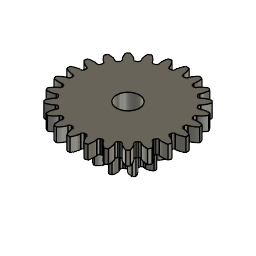
IntermediateGear1 (Autodesk Fusion 360 design; units mm, degrees)
part number: 2026-05-31-22-24-32-655
Autodesk Fusion 360 part; units mm, degrees
sketch "Base Circle" plane through (0, 0, 0) normal (0, 0, 1) x (1, 0, 0)
  circle A0 centre (0, 0) radius 1.9215
  circle A1 centre (0, 0) radius 1.25
  dimension "d49" = 2.5
  measures "d49" diameter of A1
extrude "Extrude9" add sketch "Base Circle" along normal blind 10 makes body 1
sketch "Gear Tooth" plane through (0, 0, 0) normal (0, 0, 1) x (1, 0, 0)
  spline S0 degree 5 poles (2.3146, -0.402) (2.3164, -0.4024) (2.3202, -0.403) (2.3258, -0.4036) (2.3334, -0.4042) (2.3429, -0.4044) (2.3525, -0.4042) (2.3621, -0.4039) (2.3717, -0.4033) (2.3814, -0.4027) (2.3911, -0.4021) (2.4007, -0.4013) (2.4104, -0.4003) (2.4202, -0.3992) (2.4299, -0.3979) (2.4396, -0.3964) (2.4494, -0.3947) (2.4592, -0.393) (2.469, -0.3911) (2.4788, -0.3892) (2.4886, -0.3871) (2.4984, -0.3849) (2.5082, -0.3826) (2.518, -0.3802) (2.5279, -0.3777) (2.5377, -0.3751) (2.5476, -0.3723) (2.5574, -0.3695) (2.5673, -0.3665) (2.5771, -0.3634) (2.587, -0.3603) (2.5968, -0.357) (2.6067, -0.3537) (2.6166, -0.3503) (2.6264, -0.3467) (2.6363, -0.3431) (2.6462, -0.3393) (2.656, -0.3355) (2.6659, -0.3316) (2.6757, -0.3276) (2.6856, -0.3235) (2.6954, -0.3193) (2.7053, -0.315) (2.7151, -0.3106) (2.7249, -0.3061) (2.7348, -0.3016) (2.7446, -0.2969) (2.7544, -0.2922) (2.7642, -0.2874) (2.774, -0.2825) (2.7838, -0.2775) (2.7936, -0.2724) (2.8034, -0.2673) (2.8131, -0.262) (2.8229, -0.2567) (2.8327, -0.2513) (2.8424, -0.2458) (2.8521, -0.2402) (2.8618, -0.2346) (2.8715, -0.2288) (2.8812, -0.223) (2.8909, -0.2171) (2.9006, -0.2111) (2.9102, -0.2051) (2.9199, -0.1989) (2.9295, -0.1927) (2.9391, -0.1864) (2.9487, -0.18) (2.9583, -0.1735) (2.9678, -0.167) (2.9774, -0.1604) (2.985, -0.155) (2.9907, -0.151) (2.9945, -0.1482) (2.9964, -0.1469) knots 0 0 0 0 0 0 0.01428571 0.02857143 0.04285714 0.05714286 0.07142857 0.08571429 0.1 0.11428571 0.12857143 0.14285714 0.15714286 0.17142857 0.18571429 0.2 0.21428571 0.22857143 0.24285714 0.25714286 0.27142857 0.28571429 0.3 0.31428571 0.32857143 0.34285714 0.35714286 0.37142857 0.38571429 0.4 0.41428571 0.42857143 0.44285714 0.45714286 0.47142857 0.48571429 0.5 0.51428571 0.52857143 0.54285714 0.55714286 0.57142857 0.58571429 0.6 0.61428571 0.62857143 0.64285714 0.65714286 0.67142857 0.68571429 0.7 0.71428571 0.72857143 0.74285714 0.75714286 0.77142857 0.78571429 0.8 0.81428571 0.82857143 0.84285714 0.85714286 0.87142857 0.88571429 0.9 0.91428571 0.92857143 0.94285714 0.95714286 0.97142857 0.98571429 1 1 1 1 1 1
  spline S1 degree 5 poles (2.3146, 0.402) (2.3164, 0.4024) (2.3202, 0.403) (2.3258, 0.4036) (2.3334, 0.4042) (2.3429, 0.4044) (2.3525, 0.4042) (2.3621, 0.4039) (2.3717, 0.4033) (2.3814, 0.4027) (2.3911, 0.4021) (2.4007, 0.4013) (2.4104, 0.4003) (2.4202, 0.3992) (2.4299, 0.3979) (2.4396, 0.3964) (2.4494, 0.3947) (2.4592, 0.393) (2.469, 0.3911) (2.4788, 0.3892) (2.4886, 0.3871) (2.4984, 0.3849) (2.5082, 0.3826) (2.518, 0.3802) (2.5279, 0.3777) (2.5377, 0.3751) (2.5476, 0.3723) (2.5574, 0.3695) (2.5673, 0.3665) (2.5771, 0.3634) (2.587, 0.3603) (2.5968, 0.357) (2.6067, 0.3537) (2.6166, 0.3503) (2.6264, 0.3467) (2.6363, 0.3431) (2.6462, 0.3393) (2.656, 0.3355) (2.6659, 0.3316) (2.6757, 0.3276) (2.6856, 0.3235) (2.6954, 0.3193) (2.7053, 0.315) (2.7151, 0.3106) (2.7249, 0.3061) (2.7348, 0.3016) (2.7446, 0.2969) (2.7544, 0.2922) (2.7642, 0.2874) (2.774, 0.2825) (2.7838, 0.2775) (2.7936, 0.2724) (2.8034, 0.2673) (2.8131, 0.262) (2.8229, 0.2567) (2.8327, 0.2513) (2.8424, 0.2458) (2.8521, 0.2402) (2.8618, 0.2346) (2.8715, 0.2288) (2.8812, 0.223) (2.8909, 0.2171) (2.9006, 0.2111) (2.9102, 0.2051) (2.9199, 0.1989) (2.9295, 0.1927) (2.9391, 0.1864) (2.9487, 0.18) (2.9583, 0.1735) (2.9678, 0.167) (2.9774, 0.1604) (2.985, 0.155) (2.9907, 0.151) (2.9945, 0.1482) (2.9964, 0.1469) knots 0 0 0 0 0 0 0.01428571 0.02857143 0.04285714 0.05714286 0.07142857 0.08571429 0.1 0.11428571 0.12857143 0.14285714 0.15714286 0.17142857 0.18571429 0.2 0.21428571 0.22857143 0.24285714 0.25714286 0.27142857 0.28571429 0.3 0.31428571 0.32857143 0.34285714 0.35714286 0.37142857 0.38571429 0.4 0.41428571 0.42857143 0.44285714 0.45714286 0.47142857 0.48571429 0.5 0.51428571 0.52857143 0.54285714 0.55714286 0.57142857 0.58571429 0.6 0.61428571 0.62857143 0.64285714 0.65714286 0.67142857 0.68571429 0.7 0.71428571 0.72857143 0.74285714 0.75714286 0.77142857 0.78571429 0.8 0.81428571 0.82857143 0.84285714 0.85714286 0.87142857 0.88571429 0.9 0.91428571 0.92857143 0.94285714 0.95714286 0.97142857 0.98571429 1 1 1 1 1 1
  arc A0 (2.9964, -0.1469) -> (2.9964, 0.1469) centre (0, 0) ccw
  line L0 (1.8833, -0.3271) -> (2.3146, -0.402)
  line L1 (1.8833, 0.3271) -> (2.3146, 0.402)
  line L2 (1.8833, -0.3271) -> (1.8833, 0.3271)
  point P0 (2.3614, -0.4039)
  point P1 (2.4092, -0.4004)
  point P2 (2.4574, -0.3933)
  point P3 (2.5061, -0.3831)
  point P4 (2.555, -0.3701)
  point P5 (2.6041, -0.3546)
  point P6 (2.6534, -0.3365)
  point P7 (2.7027, -0.3161)
  point P8 (2.752, -0.2934)
  point P9 (2.8012, -0.2684)
  point P10 (2.8504, -0.2412)
  point P11 (2.8993, -0.2119)
  point P12 (2.948, -0.1804)
  point P13 (2.3614, 0.4039)
  point P14 (2.4092, 0.4004)
  point P15 (2.4574, 0.3933)
  point P16 (2.5061, 0.3831)
  point P17 (2.555, 0.3701)
  point P18 (2.6041, 0.3546)
  point P19 (2.6534, 0.3365)
  point P20 (2.7027, 0.3161)
  point P21 (2.752, 0.2934)
  point P22 (2.8012, 0.2684)
  point P23 (2.8504, 0.2412)
  point P24 (2.8993, 0.2119)
  point P25 (2.948, 0.1804)
extrude "Extrude10" add sketch "Gear Tooth" along normal blind 10 bodies 1
fillet "Fillet4" radius 0.2 2 edges at (1.8932, -0.3288, 5) (1.8932, 0.3288, 5) on bodies 1
pattern_circular "C-Pattern4" count 10 over 360 about axis through (0, 0, 0) along (0, 0, 1) of "Extrude10", "Fillet4"
sketch "Diametrial Pitch Circle" plane through (0, 0, 0) normal (0, 0, 1) x (1, 0, 0)
  circle A0 centre (0, 0) radius 2.5 construction
extrude "Extrude11" cut 1 faces at (1.7096, 0, 10) along direction (0, 0, -1) blind 8 on bodies 1 bodies 1
sketch "Base Circle (1)" plane through (0, 0, 0) normal (0, 0, 1) x (1, 0, 0)
  circle A0 centre (0, 0) radius 5.4215
  circle A1 centre (0, 0) radius 1.25
  dimension "d50" = 2.5
  measures "d50" diameter of A1
extrude "Extrude12" add sketch "Base Circle (1)" along normal blind 10 separate body makes body 2
sketch "Gear Tooth (1)" plane through (0, 0, 0) normal (0, 0, 1) x (1, 0, 0)
  spline S0 degree 5 poles (5.62, -0.4526) (5.6225, -0.4528) (5.6274, -0.4531) (5.6349, -0.4534) (5.6449, -0.4535) (5.6574, -0.4531) (5.6699, -0.4524) (5.6824, -0.4514) (5.695, -0.4503) (5.7075, -0.4491) (5.7201, -0.4479) (5.7326, -0.4465) (5.7452, -0.445) (5.7578, -0.4434) (5.7703, -0.4415) (5.7829, -0.4395) (5.7955, -0.4374) (5.8081, -0.4351) (5.8207, -0.4328) (5.8333, -0.4303) (5.8459, -0.4278) (5.8585, -0.4252) (5.8711, -0.4224) (5.8837, -0.4196) (5.8963, -0.4166) (5.9089, -0.4135) (5.9215, -0.4104) (5.9341, -0.4071) (5.9467, -0.4038) (5.9593, -0.4003) (5.9719, -0.3968) (5.9845, -0.3932) (5.9971, -0.3895) (6.0097, -0.3857) (6.0223, -0.3819) (6.0349, -0.3779) (6.0475, -0.3739) (6.0601, -0.3697) (6.0727, -0.3655) (6.0853, -0.3613) (6.0978, -0.3569) (6.1104, -0.3525) (6.123, -0.348) (6.1356, -0.3434) (6.1481, -0.3387) (6.1607, -0.3339) (6.1732, -0.3291) (6.1858, -0.3242) (6.1983, -0.3193) (6.2109, -0.3142) (6.2234, -0.3091) (6.2359, -0.3039) (6.2485, -0.2986) (6.261, -0.2933) (6.2735, -0.2879) (6.286, -0.2824) (6.2985, -0.2769) (6.311, -0.2713) (6.3235, -0.2656) (6.336, -0.2598) (6.3485, -0.254) (6.3609, -0.2481) (6.3734, -0.2421) (6.3858, -0.2361) (6.3983, -0.23) (6.4107, -0.2239) (6.4231, -0.2176) (6.4356, -0.2113) (6.448, -0.205) (6.4604, -0.1985) (6.4728, -0.1921) (6.4827, -0.1868) (6.4901, -0.1828) (6.4951, -0.1802) (6.4975, -0.1789) knots 0 0 0 0 0 0 0.01428571 0.02857143 0.04285714 0.05714286 0.07142857 0.08571429 0.1 0.11428571 0.12857143 0.14285714 0.15714286 0.17142857 0.18571429 0.2 0.21428571 0.22857143 0.24285714 0.25714286 0.27142857 0.28571429 0.3 0.31428571 0.32857143 0.34285714 0.35714286 0.37142857 0.38571429 0.4 0.41428571 0.42857143 0.44285714 0.45714286 0.47142857 0.48571429 0.5 0.51428571 0.52857143 0.54285714 0.55714286 0.57142857 0.58571429 0.6 0.61428571 0.62857143 0.64285714 0.65714286 0.67142857 0.68571429 0.7 0.71428571 0.72857143 0.74285714 0.75714286 0.77142857 0.78571429 0.8 0.81428571 0.82857143 0.84285714 0.85714286 0.87142857 0.88571429 0.9 0.91428571 0.92857143 0.94285714 0.95714286 0.97142857 0.98571429 1 1 1 1 1 1
  spline S1 degree 5 poles (5.62, 0.4526) (5.6225, 0.4528) (5.6274, 0.4531) (5.6349, 0.4534) (5.6449, 0.4535) (5.6574, 0.4531) (5.6699, 0.4524) (5.6824, 0.4514) (5.695, 0.4503) (5.7075, 0.4491) (5.7201, 0.4479) (5.7326, 0.4465) (5.7452, 0.445) (5.7578, 0.4434) (5.7703, 0.4415) (5.7829, 0.4395) (5.7955, 0.4374) (5.8081, 0.4351) (5.8207, 0.4328) (5.8333, 0.4303) (5.8459, 0.4278) (5.8585, 0.4252) (5.8711, 0.4224) (5.8837, 0.4196) (5.8963, 0.4166) (5.9089, 0.4135) (5.9215, 0.4104) (5.9341, 0.4071) (5.9467, 0.4038) (5.9593, 0.4003) (5.9719, 0.3968) (5.9845, 0.3932) (5.9971, 0.3895) (6.0097, 0.3857) (6.0223, 0.3819) (6.0349, 0.3779) (6.0475, 0.3739) (6.0601, 0.3697) (6.0727, 0.3655) (6.0853, 0.3613) (6.0978, 0.3569) (6.1104, 0.3525) (6.123, 0.348) (6.1356, 0.3434) (6.1481, 0.3387) (6.1607, 0.3339) (6.1732, 0.3291) (6.1858, 0.3242) (6.1983, 0.3193) (6.2109, 0.3142) (6.2234, 0.3091) (6.2359, 0.3039) (6.2485, 0.2986) (6.261, 0.2933) (6.2735, 0.2879) (6.286, 0.2824) (6.2985, 0.2769) (6.311, 0.2713) (6.3235, 0.2656) (6.336, 0.2598) (6.3485, 0.254) (6.3609, 0.2481) (6.3734, 0.2421) (6.3858, 0.2361) (6.3983, 0.23) (6.4107, 0.2239) (6.4231, 0.2176) (6.4356, 0.2113) (6.448, 0.205) (6.4604, 0.1985) (6.4728, 0.1921) (6.4827, 0.1868) (6.4901, 0.1828) (6.4951, 0.1802) (6.4975, 0.1789) knots 0 0 0 0 0 0 0.01428571 0.02857143 0.04285714 0.05714286 0.07142857 0.08571429 0.1 0.11428571 0.12857143 0.14285714 0.15714286 0.17142857 0.18571429 0.2 0.21428571 0.22857143 0.24285714 0.25714286 0.27142857 0.28571429 0.3 0.31428571 0.32857143 0.34285714 0.35714286 0.37142857 0.38571429 0.4 0.41428571 0.42857143 0.44285714 0.45714286 0.47142857 0.48571429 0.5 0.51428571 0.52857143 0.54285714 0.55714286 0.57142857 0.58571429 0.6 0.61428571 0.62857143 0.64285714 0.65714286 0.67142857 0.68571429 0.7 0.71428571 0.72857143 0.74285714 0.75714286 0.77142857 0.78571429 0.8 0.81428571 0.82857143 0.84285714 0.85714286 0.87142857 0.88571429 0.9 0.91428571 0.92857143 0.94285714 0.95714286 0.97142857 0.98571429 1 1 1 1 1 1
  arc A0 (6.4975, -0.1789) -> (6.4975, 0.1789) centre (0, 0) ccw
  line L0 (5.394, -0.4344) -> (5.62, -0.4526)
  line L1 (5.394, 0.4344) -> (5.62, 0.4526)
  line L2 (5.394, -0.4344) -> (5.394, 0.4344)
  point P0 (5.6818, -0.4514)
  point P1 (5.7441, -0.4451)
  point P2 (5.8065, -0.4354)
  point P3 (5.8692, -0.4228)
  point P4 (5.932, -0.4076)
  point P5 (5.9948, -0.3902)
  point P6 (6.0578, -0.3705)
  point P7 (6.1207, -0.3488)
  point P8 (6.1837, -0.325)
  point P9 (6.2466, -0.2994)
  point P10 (6.3095, -0.2719)
  point P11 (6.3723, -0.2427)
  point P12 (6.435, -0.2116)
  point P13 (5.6818, 0.4514)
  point P14 (5.7441, 0.4451)
  point P15 (5.8065, 0.4354)
  point P16 (5.8692, 0.4228)
  point P17 (5.932, 0.4076)
  point P18 (5.9948, 0.3902)
  point P19 (6.0578, 0.3705)
  point P20 (6.1207, 0.3488)
  point P21 (6.1837, 0.325)
  point P22 (6.2466, 0.2994)
  point P23 (6.3095, 0.2719)
  point P24 (6.3723, 0.2427)
  point P25 (6.435, 0.2116)
extrude "Extrude13" add sketch "Gear Tooth (1)" along normal blind 10 bodies 2
fillet "Fillet5" radius 0.2 2 edges at (5.404, -0.4352, 5) (5.404, 0.4352, 5) on bodies 2
pattern_circular "C-Pattern5" count 24 over 360 about axis through (0, 0, 0) along (0, 0, 1) of "Extrude13", "Fillet5"
sketch "Diametrial Pitch Circle (1)" plane through (0, 0, 0) normal (0, 0, 1) x (1, 0, 0)
  circle A0 centre (0, 0) radius 6 construction
move_body "Move2" bodies 2 to x (1, 0, 0) y (0, 1, 0) z (0, 0, 1) at (0, 0, 2)
extrude "Extrude14" cut 1 faces at (4.0113, 0, 12) along direction (0, 0, -1) blind 7 on bodies 2 bodies 2
extrude "Extrude15" cut 1 faces at (4.0113, 0, 2) along direction (0, 0, 1) blind 1.5 on bodies 2 bodies 2
extrude "Extrude16" add 1 faces at (1.7096, 0, 2) along direction (0, 0, 1) blind 2.1 on bodies 1 bodies 1 2
named bodies: "Spur Gear (10 teeth)", "Spur Gear (24 teeth)"
